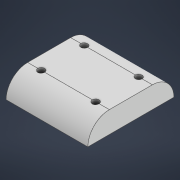
# Autodesk Inventor part: jump
Saved by Autodesk Inventor 2022 (Build 260153000, 153)
## iProperties
Created: 2022-01-27
Part Number: jump
Material: 一般
Document SubType Name: Modeling
Designer: shiokaze
Density: 1 g/cm^3
Appearance: 既定
Author: shiokaze
Autodesk Inventor part; units mm, degrees
ref_plane "YZ Plane" through (0, 0, 0) normal (1, 0, 0) x (0, 1, 0)
ref_plane "XZ Plane" through (0, 0, 0) normal (0, 1, 0) x (-1, 0, 0)
ref_plane "XY Plane" through (0, 0, 0) normal (0, 0, 1) x (1, 0, 0)
sketch "スケッチ1" plane through (0, 0, 0) normal (0, 1, 0) x (-1, 0, 0)
  line L0 (9.5, -10) -> (-9.5, -10)
  line L1 (-9.5, -10) -> (-9.5, 10)
  line L2 (-9.5, 10) -> (9.5, 10)
  line L3 (9.5, 10) -> (9.5, -10)
  line L4 (9.5, -10) -> (-9.5, 10) construction
  point P0 (0, 0)
  point P1 (0, 0)
  dimension "d0" = 19
  dimension "d1" = 20
  constraints: 10 end point, 2 parallel, 1 coincident, 1 horizontal, 1 midpoint, 1 perpendicular
  measures "d0" distance of L1.end L2.end
  measures "d1" distance of L0.end L1.end
extrude "押し出し1" add sketch "スケッチ1" along normal blind 5
sketch "スケッチ3" plane through (0, 0, 0) normal (0, -1, 0) x (1, 0, 0)
  line L0 (-9.5, 10) -> (9.5, 10) projected
  line L1 (-9.5, -10) -> (-9.5, 10) projected
  line L2 (9.5, -10) -> (-9.5, -10) projected
  line L3 (9.5, 10) -> (9.5, -10) projected
  line L4 (-9.5, 0) -> (9.5, 0)
  line L5 (-9.5, 10) -> (9.5, 10) projected
  line L6 (0, 10) -> (0, -10)
  line L7 (0, 2.5) -> (-3.1667, 2.5)
  line L8 (-3.1667, 2.5) -> (-3.1667, 7.5)
  line L9 (-3.1667, 7.5) -> (0, 7.5)
  line L10 (0, 2.5) -> (3.1667, 2.5)
  line L11 (3.1667, 2.5) -> (3.1667, 7.5)
  line L12 (3.1667, 7.5) -> (0, 7.5)
  line L13 (0, -2.5) -> (-3.1667, -2.5)
  line L14 (-3.1667, -2.5) -> (-3.1667, -7.5)
  line L15 (-3.1667, -7.5) -> (0, -7.5)
  line L16 (3.1667, -2.5) -> (3.1667, -7.5)
  line L17 (0, -2.5) -> (3.1667, -2.5)
  line L18 (3.1667, -7.5) -> (0, -7.5)
  point P0 (0, 0)
  point P1 (0, 0)
  dimension "d8" = 3.1667
  dimension "d9" = 2.5
  dimension "d10" = 5
  constraints: 28 end point, 8 symmetric about line, 4 midpoint, 2 point on line, 1 coincident, 1 horizontal, 1 parallel, 1 perpendicular
  measures "d8" distance of L7.start L7.end
  measures "d9" distance between parallel lines of L4 L7
  measures "d10" distance of L7.end L8.end
extrude "押し出し2" add sketch "スケッチ3" along normal blind 1.6 contours L12 L11 L10 L6 | L6 L7 L8 L9 | L17 L16 L18 L6 | L6 L15 L14 L13
sketch "スケッチ4" plane through (0, -1.6, 0) normal (0, -1, 0) x (1, 0, 0)
  line L0 (3.1667, 2.5) -> (3.1667, 7.5) projected
  line L1 (-3.1667, 7.5) -> (-3.1667, 2.5) projected
  line L2 (-3.1667, -2.5) -> (-3.1667, -7.5) projected
  line L3 (3.1667, -7.5) -> (3.1667, -2.5) projected
  line L4 (3.1667, 7.5) -> (3.1667, 2.5) construction
  line L5 (3.1667, 5) -> (6.3333, 5) construction
  line L6 (6.3333, 5) -> (9.5, 5) construction
  line L7 (9.5, 10) -> (9.5, -10) construction
  line L8 (9.5, 0) -> (-9.5, 0)
  line L9 (-9.5, -10) -> (-9.5, 10) projected
  line L10 (3.1667, 2.5) -> (-3.1667, 2.5) projected
  line L11 (0, 2.5) -> (0, -2.5)
  point P0 (0, 0)
  point P1 (6.3333, -5)
  point P2 (-6.3333, 5)
  point P3 (-6.3333, -5)
  constraints: 8 end point, 4 midpoint, 3 symmetric about line, 2 horizontal, 1 collinear, 1 point on line, 1 vertical
hole "穴1" at (6.3333, -1.6, 5) at (6.3333, -1.6, -5) at (-6.3333, -1.6, 5) at (-6.3333, -1.6, -5) direction (0, 1, 0) diameter 1.567 end through all thread size "M2x0.4" class "6H" standard "ISO Metric profile"
fillet "フィレット1" radius 1.5 8 edges at (3.1667, -0.8, 2.5) (3.1667, -0.8, 7.5) (-3.1667, -0.8, 7.5) (-3.1667, -0.8, 2.5) (3.1667, -0.8, -2.5) (3.1667, -0.8, -7.5) (-3.1667, -0.8, -7.5) (-3.1667, -0.8, -2.5)
fillet "フィレット2" radius 5 2 edges at (0, 5, -10) (0, 5, 10)
